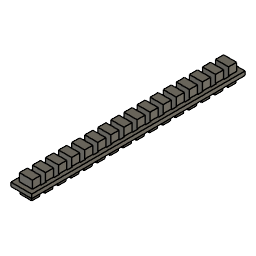
spacer (Autodesk Fusion 360 design; units mm, degrees)
Autodesk Fusion 360 part; units mm, degrees
sketch "スケッチ1" plane through (0, 0, 0) normal (0, 0, 1) x (1, 0, 0)
  line L0 (0, 0) -> (5, 0)
  line L1 (5, 0) -> (5, 78.6)
  line L2 (5, 78.6) -> (0, 78.6)
  line L3 (0, 78.6) -> (0, 0)
  line L4 (-1.5, -1.5) -> (6.5, -1.5)
  line L5 (6.5, -1.5) -> (6.5, 80.1)
  line L6 (6.5, 80.1) -> (-1.5, 80.1)
  line L7 (-1.5, 80.1) -> (-1.5, -1.5)
  line L8 (-0.25, -0.25) -> (5.25, -0.25)
  line L9 (5.25, -0.25) -> (5.25, 78.85)
  line L10 (5.25, 78.85) -> (-0.25, 78.85)
  line L11 (-0.25, 78.85) -> (-0.25, -0.25)
  line L12 (-0.25, 3.35) -> (5.25, 3.35)
  line L13 (5.25, 3.35) -> (5.25, 0.25)
  line L14 (5.25, 0.25) -> (-0.25, 0.25)
  line L15 (-0.25, 0.25) -> (-0.25, 3.35)
  line L16 (0.25, 78.35) -> (0.25, 0.25)
  line L17 (0.25, 0.25) -> (4.75, 0.25)
  line L18 (4.75, 0.25) -> (4.75, 78.35)
  line L19 (4.75, 78.35) -> (0.25, 78.35)
  line L20 (5.25, 5.25) -> (-0.25, 5.25)
  line L21 (-0.25, 8.35) -> (5.25, 8.35)
  line L22 (5.25, 10.25) -> (-0.25, 10.25)
  line L23 (-0.25, 13.35) -> (5.25, 13.35)
  line L24 (5.25, 15.25) -> (-0.25, 15.25)
  line L25 (-0.25, 18.35) -> (5.25, 18.35)
  line L26 (5.25, 20.25) -> (-0.25, 20.25)
  line L27 (-0.25, 23.35) -> (5.25, 23.35)
  line L28 (5.25, 25.25) -> (-0.25, 25.25)
  line L29 (-0.25, 28.35) -> (5.25, 28.35)
  line L30 (5.25, 30.25) -> (-0.25, 30.25)
  line L31 (-0.25, 33.35) -> (5.25, 33.35)
  line L32 (5.25, 35.25) -> (-0.25, 35.25)
  line L33 (-0.25, 38.35) -> (5.25, 38.35)
  line L34 (5.25, 40.25) -> (-0.25, 40.25)
  line L35 (-0.25, 43.35) -> (5.25, 43.35)
  line L36 (5.25, 45.25) -> (-0.25, 45.25)
  line L37 (-0.25, 48.35) -> (5.25, 48.35)
  line L38 (5.25, 50.25) -> (-0.25, 50.25)
  line L39 (-0.25, 53.35) -> (5.25, 53.35)
  line L40 (5.25, 55.25) -> (-0.25, 55.25)
  line L41 (-0.25, 58.35) -> (5.25, 58.35)
  line L42 (5.25, 60.25) -> (-0.25, 60.25)
  line L43 (-0.25, 63.35) -> (5.25, 63.35)
  line L44 (5.25, 65.25) -> (-0.25, 65.25)
  line L45 (-0.25, 68.35) -> (5.25, 68.35)
  line L46 (5.25, 70.25) -> (-0.25, 70.25)
  line L47 (-0.25, 73.35) -> (5.25, 73.35)
  line L48 (5.25, 75.25) -> (-0.25, 75.25)
  line L49 (-0.25, 78.35) -> (5.25, 78.35)
  line L50 (5, 78.6) -> (5.25, 78.6)
  line L51 (5, 78.6) -> (5, 78.85)
  line L52 (0, 78.6) -> (0, 78.85)
  line L53 (0, 78.6) -> (-0.25, 78.6)
  line L54 (5, 0) -> (5, -0.25)
  line L55 (5, 0) -> (5.25, 0)
  line L56 (0, 0) -> (-0.25, 0)
  line L57 (0, 0) -> (0, -0.25)
  dimension "d1" = 5
  dimension "d2" = 78.6
  dimension "d3" = 1.5
  dimension "d4" = 0.25
  dimension "d5" = 3.1
  dimension "d7" = -0.25
  dimension "d8" = 0.25
  dimension "d11" = 0
  dimension "d12" = 75
  constraint horizontal L0
  constraint vertical L1
  constraint horizontal L2
  constraint vertical L3
  constraint coincident L0.start L3.end
  constraint horizontal L12
  constraint vertical L13
  constraint horizontal L14
  constraint vertical L15
  constraint coincident L9 L13.end
  constraint coincident L11 L12.start
  constraint coincident L9 L50.end
  constraint perpendicular L9 L50
  constraint coincident L10 L51.end
  constraint perpendicular L10 L51
  constraint coincident L10 L52.end
  constraint perpendicular L10 L52
  constraint coincident L11 L53.end
  constraint perpendicular L11 L53
  constraint coincident L8 L54.end
  constraint perpendicular L8 L54
  constraint coincident L9 L55.end
  constraint perpendicular L9 L55
  constraint coincident L11 L56.end
  constraint perpendicular L11 L56
  constraint coincident L8 L57.end
  constraint perpendicular L8 L57
  measures "d1" distance of L0.start L0.end
  measures "d2" distance of L0.start L2.end
  measures "d5" distance of L12 L14
  measures "d8" distance of L0 L14
extrude "押し出し6" add sketch "スケッチ1" against normal blind 1.5 contours L0 L1 L3 L14 L17 | L3 L11 L14 L56 | L8 L11 L56 L57 | L0 L8 L54 L57 | L8 L9 L54 L55 | L1 L9 L14 L55 | L3 L11 L12 L14 L15 | L3 L12 L14 L16 | L1 L12 L14 L18 | L1 L9 L12 L13 L14 | L12 L14 L16 L17 L18 | L3 L11 L20 L21 | L3 L16 L20 L21 | L1 L18 L20 L21 | L1 L9 L20 L21 | L16 L18 L20 L21 | L3 L11 L22 L23 | L3 L16 L22 L23 | L1 L18 L22 L23 | L1 L9 L22 L23 | L16 L18 L22 L23 | L3 L11 L24 L25 | L3 L16 L24 L25 | L1 L18 L24 L25 | L1 L9 L24 L25 | L16 L18 L24 L25 | L3 L11 L26 L27 | L3 L16 L26 L27 | L1 L18 L26 L27 | L1 L9 L26 L27 | L16 L18 L26 L27 | L3 L11 L28 L29 | L3 L16 L28 L29 | L1 L18 L28 L29 | L1 L9 L28 L29 | L16 L18 L28 L29 | L3 L11 L30 L31 | L3 L16 L30 L31 | L1 L18 L30 L31 | L1 L9 L30 L31 | L16 L18 L30 L31 | L3 L11 L32 L33 | L3 L16 L32 L33 | L1 L18 L32 L33 | L1 L9 L32 L33 | L16 L18 L32 L33 | L3 L11 L34 L35 | L3 L16 L34 L35 | L1 L18 L34 L35 | L1 L9 L34 L35 | L16 L18 L34 L35 | L3 L11 L36 L37 | L3 L16 L36 L37 | L1 L18 L36 L37 | L1 L9 L36 L37 | L16 L18 L36 L37 | L3 L11 L38 L39 | L3 L16 L38 L39 | L1 L18 L38 L39 | L1 L9 L38 L39 | L16 L18 L38 L39 | L3 L11 L40 L41 | L3 L16 L40 L41 | L1 L18 L40 L41 | L1 L9 L40 L41 | L16 L18 L40 L41 | L3 L11 L42 L43 | L3 L16 L42 L43 | L1 L18 L42 L43 | L1 L9 L42 L43 | L16 L18 L42 L43 | L3 L11 L44 L45 | L3 L16 L44 L45 | L1 L18 L44 L45 | L1 L9 L44 L45 | L16 L18 L44 L45 | L3 L11 L46 L47 | L3 L16 L46 L47 | L1 L18 L46 L47 | L1 L9 L46 L47 | L16 L18 L46 L47 | L3 L11 L48 L49 | L3 L16 L48 L49 | L1 L18 L48 L49 | L1 L9 L48 L49 | L3 L11 L49 L53 | L1 L2 L3 L19 L49 | L16 L18 L19 L48 L49 | L1 L9 L49 L50 | L2 L10 L51 L52 | L10 L11 L52 L53 | L9 L10 L50 L51 | L4 L5 L6 L7
extrude "押し出し7" add sketch "スケッチ1" against normal blind 4 contours L12 L14 L16 L17 L18 | L16 L18 L20 L21 | L16 L18 L22 L23 | L16 L18 L24 L25 | L16 L18 L26 L27 | L16 L18 L28 L29 | L16 L18 L30 L31 | L16 L18 L32 L33 | L16 L18 L34 L35 | L16 L18 L36 L37 | L16 L18 L38 L39 | L16 L18 L40 L41 | L16 L18 L42 L43 | L16 L18 L44 L45 | L16 L18 L46 L47 | L16 L18 L19 L48 L49
extrude "押し出し8" add sketch "スケッチ1" along normal blind 3 contours L3 L12 L14 L16 | L1 L12 L14 L18 | L12 L14 L16 L17 L18 | L3 L16 L20 L21 | L1 L18 L20 L21 | L16 L18 L20 L21 | L3 L16 L22 L23 | L1 L18 L22 L23 | L16 L18 L22 L23 | L3 L16 L24 L25 | L1 L18 L24 L25 | L16 L18 L24 L25 | L3 L16 L26 L27 | L1 L18 L26 L27 | L16 L18 L26 L27 | L3 L16 L28 L29 | L1 L18 L28 L29 | L16 L18 L28 L29 | L3 L16 L30 L31 | L1 L18 L30 L31 | L16 L18 L30 L31 | L3 L16 L32 L33 | L1 L18 L32 L33 | L16 L18 L32 L33 | L3 L16 L34 L35 | L1 L18 L34 L35 | L16 L18 L34 L35 | L3 L16 L36 L37 | L1 L18 L36 L37 | L16 L18 L36 L37 | L3 L16 L38 L39 | L1 L18 L38 L39 | L16 L18 L38 L39 | L3 L16 L40 L41 | L1 L18 L40 L41 | L16 L18 L40 L41 | L3 L16 L42 L43 | L1 L18 L42 L43 | L16 L18 L42 L43 | L3 L16 L44 L45 | L1 L18 L44 L45 | L16 L18 L44 L45 | L3 L16 L46 L47 | L1 L18 L46 L47 | L16 L18 L46 L47 | L3 L16 L48 L49 | L1 L18 L48 L49 | L16 L18 L19 L48 L49
extrude "押し出し1" [rolled back] along distance -1.5 taper angle 0
extrude "押し出し2" [rolled back] along distance -4 taper angle 0
extrude "押し出し3" [rolled back] along distance 3 taper angle 0
extrude "押し出し4" [rolled back] along distance 3 taper angle 0
combine "結合1" [rolled back]
extrude "押し出し5" [rolled back] along distance 7 taper angle 0
